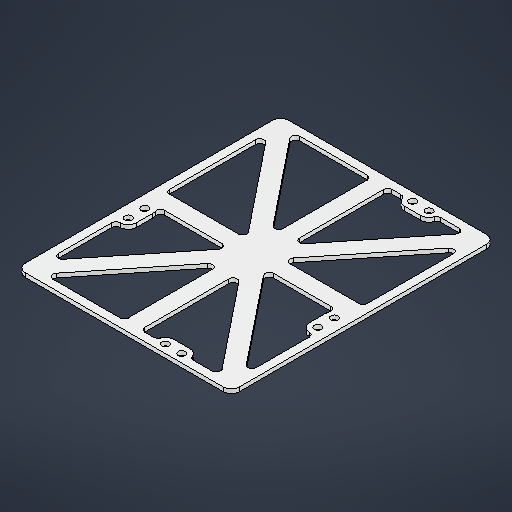
# Autodesk Inventor part: PLATE_LEFT
Saved by Autodesk Inventor 2026.1 (Build 301233020, 233B)
## iProperties
Created: 2026-03-30
Part Number: PLATE_LEFT
Material: Aluminum 6061
Document SubType Name: Sheet Metal
Designer: Owen L
Density: 2.7 g/cm^3
Sheet Metal Rule: Default
Appearance: Aluminum - Flat
Mass: 67.1671 g
Surface Area: 251.931 cm^2
Volume: 24.8767 cm^3
Author: Owen L
Autodesk Inventor part; units mm, degrees
ref_plane "YZ Plane" through (0, 0, 0) normal (1, 0, 0) x (0, 1, 0)
ref_plane "XZ Plane" through (0, 0, 0) normal (0, 1, 0) x (-1, 0, 0)
ref_plane "XY Plane" through (0, 0, 0) normal (0, 0, 1) x (1, 0, 0)
sketch "Sketch1" plane through (0, 0, 0) normal (0, 1, 0) x (-1, 0, 0)
  line L0 (-82.55, 101.6) -> (82.55, 101.6)
  line L1 (82.55, 101.6) -> (82.55, -101.6)
  line L2 (82.55, -101.6) -> (-82.55, -101.6)
  line L3 (-82.55, -101.6) -> (-82.55, 101.6)
  line L4 (-82.55, 101.6) -> (82.55, -101.6) construction
  line L5 (82.55, 101.6) -> (-82.55, -101.6) construction
  point P0 (0, 0)
  dimension "d0" = 165.1
  dimension "d1" = 203.2
  measures "d0" distance of L1.end L2.end
  measures "d1" distance of L0.end L1.end
extrude "Plate1" add sketch "Sketch1" along normal blind 3.175
sketch "Sketch2" plane through (0, 3.175, 0) normal (0, 1, 0) x (1, 0, 0)
  line L0 (82.55, 101.6) -> (82.55, -101.6) projected
  line L1 (82.55, -101.6) -> (-82.55, -101.6) projected
  line L2 (-82.55, 101.6) -> (82.55, 101.6) projected
  line L3 (-82.55, -101.6) -> (-82.55, 101.6) projected
  point P0 (0, 0)
  point P1 (25.4, -95.25)
  point P2 (38.1, -95.25)
  point P3 (-73.025, -12.7)
  point P4 (-73.025, -25.4)
  point P5 (25.4, 95.25)
  point P6 (38.1, 95.25)
  point P7 (73.025, -12.7)
  point P8 (73.025, -25.4)
  dimension "d3" = 12.7
  dimension "d4" = 44.45
  dimension "d5" = 6.35
  dimension "d6" = 12.7
  dimension "d7" = 114.3
  dimension "d8" = 9.525
  dimension "d9" = 12.7
  dimension "d10" = 6.35
  dimension "d11" = 44.45
  dimension "d12" = 9.525
  constraints: 4 horizontal alignment, 2 vertical alignment
  measures "d3" distance of point (25.4, -95.25) point (38.1, -95.25)
  measures "d4" distance from line of L0 point (38.1, -95.25)
  measures "d5" distance from line of L1 point (38.1, -95.25)
  measures "d6" distance of point (-73.025, -25.4) point (-73.025, -12.7)
  measures "d7" distance from line of L2 point (-73.025, -12.7)
  measures "d8" distance from line of L3 point (-73.025, -12.7)
  measures "d9" distance of point (25.4, 95.25) point (38.1, 95.25)
  measures "d10" distance from line of L2 point (38.1, 95.25)
  measures "d11" distance from line of L0 point (38.1, 95.25)
  measures "d12" distance from line of L0 point (73.025, -12.7)
hole "Hole1" at (25.4, 3.175, 95.25) at (38.1, 3.175, 95.25) at (-73.025, 3.175, 12.7) at (-73.025, 3.175, 25.4) at (25.4, 3.175, -95.25) at (38.1, 3.175, -95.25) at (73.025, 3.175, 12.7) at (73.025, 3.175, 25.4) direction (0, -1, 0) diameter 5.6134 end through all clearance for "Flat Head Machine Screw (82)" size "#10" standard "Ansi Unified Screw Threads"
fillet "Corner Round1" radius 6.35 4 edges at (82.55, 1.5875, -101.6) (-82.55, 1.5875, -101.6) (-82.55, 1.5875, 101.6) (82.55, 1.5875, 101.6)
sketch "Sketch3" plane through (0, 3.175, 0) normal (0, 1, 0) x (1, 0, 0)
  circle A0 centre (73.025, -25.4) radius 2.8067 projected
  circle A1 centre (73.025, -12.7) radius 2.8067 projected
  circle A2 centre (38.1, 95.25) radius 2.8067 projected
  circle A3 centre (25.4, 95.25) radius 2.8067 projected
  circle A4 centre (-73.025, -25.4) radius 2.8067 projected
  circle A5 centre (-73.025, -12.7) radius 2.8067 projected
  circle A6 centre (38.1, -95.25) radius 2.8067 projected
  circle A7 centre (25.4, -95.25) radius 2.8067 projected
  arc A8 (76.2, -101.6) -> (82.55, -95.25) centre (76.2, -95.25) ccw projected
  line L0 (82.55, 95.25) -> (82.55, -95.25) projected
  arc A9 (82.55, 95.25) -> (76.2, 101.6) centre (76.2, 95.25) ccw projected
  line L1 (-76.2, 101.6) -> (76.2, 101.6) projected
  arc A10 (-76.2, 101.6) -> (-82.55, 95.25) centre (-76.2, 95.25) ccw projected
  line L2 (-82.55, -95.25) -> (-82.55, 95.25) projected
  arc A11 (-82.55, -95.25) -> (-76.2, -101.6) centre (-76.2, -95.25) ccw projected
  line L3 (76.2, -101.6) -> (-76.2, -101.6) projected
  line L4 (76.2, 95.25) -> (76.2, -95.25)
  line L5 (76.2, -95.25) -> (-76.2, -95.25)
  line L6 (-76.2, -95.25) -> (-76.2, 95.25)
  line L7 (-76.2, 95.25) -> (76.2, 95.25)
  circle A12 centre (25.4, 95.25) radius 6.35
  circle A13 centre (38.1, 95.25) radius 6.35
  circle A14 centre (73.025, -12.7) radius 6.35
  circle A15 centre (73.025, -25.4) radius 6.35
  circle A16 centre (-73.025, -12.7) radius 6.35
  circle A17 centre (-73.025, -25.4) radius 6.35
  circle A18 centre (25.4, -95.25) radius 6.35
  circle A19 centre (38.1, -95.25) radius 6.35
  line L8 (-66.675, -12.7) -> (-66.675, -25.4)
  line L9 (25.4, -88.9) -> (38.1, -88.9)
  line L10 (66.675, -25.4) -> (66.675, -12.7)
  line L11 (25.4, 88.9) -> (38.1, 88.9)
  arc A20 (76.2, -101.6) -> (82.55, -95.25) centre (76.2, -95.25) ccw projected
  line L12 (-76.2, 95.25) -> (76.2, -95.25) construction
  line L13 (-81.1585, 91.2832) -> (71.2415, -99.2168)
  line L14 (81.1585, -91.2832) -> (-71.2415, 99.2168)
  arc A21 (-71.2415, 99.2168) -> (-81.1585, 91.2832) centre (-76.2, 95.25) ccw
  arc A22 (71.2415, -99.2168) -> (81.1585, -91.2832) centre (76.2, -95.25) ccw
  line L15 (76.2, 95.25) -> (-76.2, -95.25) construction
  line L16 (71.2415, 99.2168) -> (-81.1585, -91.2832)
  line L17 (-71.2415, -99.2168) -> (81.1585, 91.2832)
  arc A23 (81.1585, 91.2832) -> (71.2415, 99.2168) centre (76.2, 95.25) ccw
  arc A24 (-81.1585, -91.2832) -> (-71.2415, -99.2168) centre (-76.2, -95.25) ccw
  line L18 (0, -101.6) -> (0, 101.6) construction
  line L19 (6.35, -101.6) -> (6.35, 101.6)
  line L20 (-6.35, 101.6) -> (-6.35, -101.6)
  arc A25 (-6.35, -101.6) -> (6.35, -101.6) centre (0, -101.6) ccw
  arc A26 (6.35, 101.6) -> (-6.35, 101.6) centre (0, 101.6) ccw
  line L21 (82.55, 0) -> (-82.55, 0) construction
  line L22 (82.55, 6.35) -> (-82.55, 6.35)
  line L23 (-82.55, -6.35) -> (82.55, -6.35)
  arc A27 (82.55, -6.35) -> (82.55, 6.35) centre (82.55, 0) ccw
  arc A28 (-82.55, 6.35) -> (-82.55, -6.35) centre (-82.55, 0) ccw
  point P0 (0, 0)
  point P1 (0, 0)
  point P2 (0, 0)
  point P3 (13.212, 6.35)
  point P4 (76.2, 6.35)
  point P5 (76.2, 85.085)
  point P6 (76.2, -6.35)
  point P7 (13.212, -6.35)
  point P8 (76.2, -85.085)
  point P9 (76.2, -30.8993)
  point P10 (76.2, -7.2007)
  point P11 (6.35, -18.1025)
  point P12 (6.35, -95.25)
  point P13 (19.05, -95.25)
  point P14 (44.45, -95.25)
  point P15 (68.068, -95.25)
  point P16 (-76.2, -30.8993)
  point P17 (-76.2, -85.085)
  point P18 (-13.212, -6.35)
  point P19 (-76.2, -6.35)
  point P20 (-76.2, -7.2007)
  point P21 (-6.35, -95.25)
  point P22 (-6.35, -18.1025)
  point P23 (-68.068, -95.25)
  point P24 (6.35, 95.25)
  point P25 (6.35, 18.1025)
  point P26 (68.068, 95.25)
  point P27 (44.45, 95.25)
  point P28 (19.05, 95.25)
  point P29 (-6.35, 18.1025)
  point P30 (-6.35, 95.25)
  point P31 (-68.068, 95.25)
  point P32 (-76.2, 6.35)
  point P33 (-13.212, 6.35)
  point P34 (-76.2, 85.085)
  point P35 (73.025, -6.35)
  point P36 (-3.052, -6.35)
  point P37 (3.052, 6.35)
  point P38 (73.025, -19.05)
  point P39 (76.2, -19.9007)
  point P40 (76.2, -18.1993)
  point P41 (-73.025, -19.05)
  point P42 (3.052, -6.35)
  point P43 (-73.025, -6.35)
  point P44 (-3.052, 6.35)
  point P45 (-76.2, -19.9007)
  point P46 (-76.2, -18.1993)
  dimension "d21" = 6.35
  dimension "d22" = 6.35
  constraints: 48 end point, 16 point on circle, 16 tangent, 8 centre point, 6 midpoint, 4 horizontal, 4 parallel, 4 vertical, 3 equal radius, 1 perpendicular, 27 other
  measures "d21" distance between parallel lines of L1 L7
  measures "d22" radius of A27
extrude "Cut1" cut sketch "Sketch3" against normal blind 3.175 contours L7 L16 L19 A12 L11 A13 | L4 L22 L17 | L14 L7 L20 | A14 L10 A15 L4 L14 L23 | L22 L6 L13 | L16 L6 A17 L8 A16 L23 | L13 L5 A19 L9 A18 L19 | L20 L5 L17
fillet "Corner Round2" radius 3.175 30 edges at (13.212, 1.5875, 6.35) (-68.068, 1.5875, -95.25) (-76.2, 1.5875, -85.085) (-76.2, 1.5875, -6.35) (-13.212, 1.5875, -6.35) (6.35, 1.5875, -95.25) (-6.35, 1.5875, -95.25) (-6.35, 1.5875, -18.1025) (6.35, 1.5875, 95.25) (-13.212, 1.5875, 6.35) (68.068, 1.5875, 95.25) (44.45, 1.5875, 95.25) (13.212, 1.5875, -6.35) (-6.35, 1.5875, 18.1025) (19.05, 1.5875, 95.25) (76.2, 1.5875, 30.8993) (76.2, 1.5875, 85.085) (-76.2, 1.5875, 85.085) (-76.2, 1.5875, 30.8993) (6.35, 1.5875, 18.1025) (6.35, 1.5875, -18.1025) (76.2, 1.5875, -6.35) (19.05, 1.5875, -95.25) (44.45, 1.5875, -95.25) (68.068, 1.5875, -95.25) (-68.068, 1.5875, 95.25) (-6.35, 1.5875, 95.25) (76.2, 1.5875, -85.085) (-73.025, 1.5875, 6.35) (73.025, 1.5875, 6.35)
equation "\"d18\" = Thickness"
equation "\"d23\" = Thickness"
equation "\"d2\" = Thickness"
equation "\"BendRadius\" = Thickness"
equation "\"BendReliefWidth\" = Thickness"
equation "\"BendReliefDepth\" = 0.5 * Thickness"
equation "\"CornerReliefSize\" = 4 * Thickness"
equation "\"MinimumRemnant\" = 2 * Thickness"
equation "\"TransitionRadius\" = BendRadius"
equation "\"JacobiRadiusSize\" = BendRadius"
equation "\"GapSize\" = Thickness"
equation "\"Thickness\" = 3.175"
body "Solid1"
